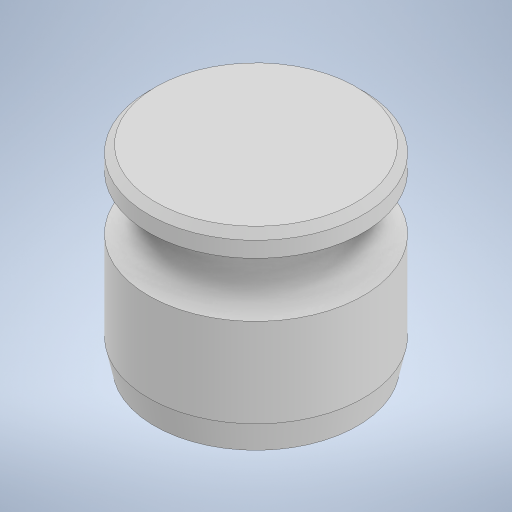
# Autodesk Inventor part: Tapita FO centelladoras
Saved by Autodesk Inventor 2024.2 (Build 282272000, 272)
## iProperties
Created: 2025-08-13
Part Number: Tapita FO centelladoras
Material: Generic
Document SubType Name: Modeling
Designer: ja.restrepo1
Density: 1 g/cm^3
Appearance: Default
Author: ja.restrepo1
Autodesk Inventor part; units mm, degrees
ref_plane "YZ Plane" through (0, 0, 0) normal (1, 0, 0) x (0, 1, 0)
ref_plane "XZ Plane" through (0, 0, 0) normal (0, 1, 0) x (-1, 0, 0)
ref_plane "XY Plane" through (0, 0, 0) normal (0, 0, 1) x (1, 0, 0)
sketch "Sketch1" plane through (0, 0, 0) normal (0, 0, 1) x (1, 0, 0)
  line L0 (-7.5, 1.8819) -> (-7.5, 8.0921)
  line L1 (-7, 13.5) -> (0, 13.5)
  line L2 (-7.5, 1.8819) -> (-7.1, 0)
  line L3 (0, 13.5) -> (0, 12)
  line L4 (0, 12) -> (-0.8, 12)
  line L5 (-6.3, 12) -> (-6.3, 7) construction
  line L6 (-6.3, 0) -> (-7.1, 0)
  arc A0 (-7.5, 8.0921) -> (-7.5, 11.9079) centre (-8.1, 10) ccw
  line L7 (-7.5, 8.0921) -> (-7.5, 11.9079) construction
  arc A1 (-7.5, 11.9079) -> (-7.5, 8.0921) centre (-8.1, 10) ccw construction
  line L8 (-7.5, 13) -> (-7, 13.5)
  line L9 (-7.5, 11.9079) -> (-7.5, 13)
  line L10 (0, -2.76) -> (0, 16.21) projected
  line L11 (-6.3, 7) -> (-0.8, 7)
  line L12 (-0.8, 7) -> (-0.8, 12)
  line L13 (-0.8, 12) -> (-6.3, 12) construction
  line L14 (-6.3, 7) -> (-6.3, 0.15)
  arc A2 (-6.2134, 0) -> (-6.3, 0.15) centre (-6.3, 0.05) ccw
  line L15 (-6.3, 0) -> (-6.2134, 0)
  arc A3 (-6.3866, 0) -> (-6.2134, 0) centre (-6.3, 0.05) ccw construction
  arc A4 (-6.3, 0.15) -> (-6.3866, 0) centre (-6.3, 0.05) ccw construction
  line L16 (-6.3, 0.15) -> (-6.3, 0) construction
  line L17 (0, 0) -> (-6.2134, 0) construction
  point P0 (-5.0852, 2.0194)
  point P1 (-0.4441, 3.0194)
  point P2 (-0.4441, 1.5194)
  point P3 (-6.1191, 3.0194)
  point P4 (0, 12.75)
  point P5 (-6.7, 0)
  point P6 (-7.5, 13.5)
  dimension "d6" = 7.5
  dimension "d8" = 13.5
  dimension "d10" = 1.5
  dimension "d11" = 6.3
  dimension "d12" = 168
  dimension "d13" = 0.8
  dimension "d14" = 4
  dimension "d15" = 10
  dimension "d16" = 1.8
  dimension "d17" = 0.5
  dimension "d18" = 0.5
  dimension "d20" = 5
  dimension "d21" = 0.8
  dimension "d25" = 0.2
  dimension "d26" = 0.05
  constraints: 34 end point, 15 perpendicular, 10 point on circle, 6 point on line, 5 centre point, 2 horizontal, 2 midpoint, 1 horizontal alignment, 1 vertical, 1 vertical alignment
  measures "d6" distance from line of L17.start L0
  measures "d8" distance between parallel lines of L6 L1
  measures "d10" distance of L1.end L3.end
  measures "d11" distance from line of L17.start L5
  measures "d12" angle of L0 L2
  measures "d13" distance of L6.start L2.end
  measures "d14" diameter of A0
  measures "d15" distance from line of L6 A0.centre
  measures "d16" distance from line of L5 A0.centre
  measures "d17" distance of L8.start point (-7.5, 13.5)
  measures "d18" distance of L1.start point (-7.5, 13.5)
  measures "d20" distance of L11.end L4.end
  measures "d21" distance from line of L17.start L12
  measures "d25" diameter of A2
  measures "d26" distance from line of A2.centre L6
revolve "Tapa FO centellador" add sketch "Sketch1" angle 360 about axis through (0, -10, 0) along (0, 1, 0)
chamfer "Chamfer1" distance 0.6 angle 45 1 edges at (0.8, 7, 0) measured on face at (1.3, 7, 0)
body "Solid1"
